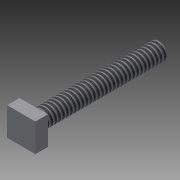
# Autodesk Inventor part: Part79
Saved by Autodesk Inventor 2015 (Build 190159000, 159)
## iProperties
Created: 2015-01-12
Part Number: Part79
Material: Generic
Document SubType Name: Modeling
Designer: mastkee16
Density: 1 g/cm^3
Appearance: Default
Author: mastkee16
Autodesk Inventor part; units mm, degrees
ref_plane "YZ Plane" through (0, 0, 0) normal (1, 0, 0) x (0, 1, 0)
ref_plane "XZ Plane" through (0, 0, 0) normal (0, 1, 0) x (-1, 0, 0)
ref_plane "XY Plane" through (0, 0, 0) normal (0, 0, 1) x (1, 0, 0)
sketch "Sketch1" plane through (0, 0, 0) normal (0, 0, 1) x (1, 0, 0)
  circle A0 centre (0, 0) radius 1.7526
  dimension "d0" = 3.5052
  constraints: 1 centre point, 1 coincident
  measures "d0" diameter of A0
extrude "Extrusion1" add sketch "Sketch1" along normal blind 25.4
sketch "Sketch2" plane through (0, 0, 25.4) normal (0, 0, 1) x (1, 0, 0)
  line L0 (-2.8702, 2.8702) -> (2.8702, 2.8702)
  line L1 (2.8702, 2.8702) -> (2.8702, -2.8702)
  line L2 (2.8702, -2.8702) -> (-2.8702, -2.8702)
  line L3 (-2.8702, -2.8702) -> (-2.8702, 2.8702)
  point P0 (0, 0)
  dimension "d3" = 5.7404
  dimension "d4" = 5.7404
  dimension "d5" = 2.8702
  dimension "d6" = 2.8702
  dimension "d7" = 2.8702
  constraints: 8 end point, 2 parallel, 1 horizontal, 1 perpendicular
  measures "d3" distance of L1.end L2.end
  measures "d4" distance of L0.end L1.end
  measures "d5" distance from line of L0 point (0, 0)
  measures "d6" distance from line of L2 point (0, 0)
  measures "d7" distance from line of L3 point (0, 0)
extrude "Extrusion2" add sketch "Sketch2" along normal blind 2.54
thread "Thread1" size "6-32 UNC" class "2A" standard "ANSI Unified Screw Threads" full length
body "Solid1"
